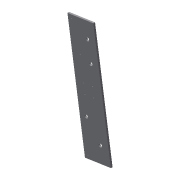
# Autodesk Inventor part: inside wall
Saved by Autodesk Inventor 2020 (Build 240168000, 168)
## iProperties
Created: 2019-10-13
Part Number: inside wall
Material: Generic
Document SubType Name: Modeling
Designer: ball
Density: 1 g/cm^3
Appearance: Default
Author: ball
Autodesk Inventor part; units mm, degrees
ref_plane "YZ Plane" through (0, 0, 0) normal (1, 0, 0) x (0, 1, 0)
ref_plane "XZ Plane" through (0, 0, 0) normal (0, 1, 0) x (-1, 0, 0)
ref_plane "XY Plane" through (0, 0, 0) normal (0, 0, 1) x (1, 0, 0)
ref_plane "Work Plane1" through (-0.0003, 0.0023, 0) normal (0, 0, 1) x (1, 0, 0)
sketch "Sketch1" plane through (-0.0003, 0.0023, 0) normal (0, 0, 1) x (1, 0, 0)
  circle A0 centre (0.0003, -0.0023) radius 6.3373 construction
  circle A1 centre (-49.0975, 326.5271) radius 6.3373 construction
  circle A2 centre (0.0003, -0.0023) radius 6.4135
  circle A3 centre (-49.0975, 326.5271) radius 6.4135
  circle A4 centre (-49.0975, 326.5271) radius 60.325 construction
  circle A5 centre (0.0003, -0.0023) radius 60.325 construction
  circle A6 centre (0.0003, -0.0023) radius 31.75 construction
  line L0 (40.3672, -54.9357) -> (-26.6702, 390.9025)
  circle A7 centre (-49.0975, 326.5271) radius 31.75 construction
  line L1 (-58.7973, -69.8464) -> (40.3672, -54.9357)
  line L2 (-125.8347, 375.9918) -> (-26.6702, 390.9025)
  circle A8 centre (-54.0299, 68.9302) radius 6.3373 construction
  circle A9 centre (-36.6118, 251.3479) radius 6.3373 construction
  circle A10 centre (-54.0299, 68.9302) radius 6.35
  circle A11 centre (-36.6118, 251.3479) radius 6.35
  line L3 (-82.6344, 131.3852) -> (-87.6899, 165.0073) construction
  line L4 (-58.7973, -69.8464) -> (-125.8347, 375.9918)
  point P0 (0.0003, -0.0023)
  dimension "d0" = 12.827
  dimension "d3" = 12.827
  dimension "d11" = 120.65
  dimension "d13" = 120.65
  dimension "d14" = 63.5
  dimension "d16" = 63.5
  dimension "d19" = 12.7
  dimension "d20" = 12.7
  constraints: 10 end point, 8 centre point, 8 coincident, 4 tangent, 3 other
  measures "d0" diameter of A2
  measures "d3" diameter of A3
  measures "d11" diameter of A4
  measures "d13" diameter of A5
  measures "d14" diameter of A6
  measures "d16" diameter of A7
  measures "d19" diameter of A10
  measures "d20" diameter of A11
extrude "Extrusion1" add sketch "Sketch1" along normal blind 6.35
sketch "Sketch2" plane through (-0.0003, 0.0023, 0) normal (0, 0, -1) x (-1, 0, 0)
  circle A0 centre (111.3879, 365.3242) radius 1.778 construction
  circle A1 centre (77.9428, 262.471) radius 1.778 construction
  circle A2 centre (31.0502, 180.1901) radius 1.778 construction
  circle A3 centre (64.857, 175.1068) radius 1.778 construction
  circle A4 centre (25.7636, 145.0307) radius 1.778 construction
  circle A5 centre (59.5704, 139.9475) radius 1.778 construction
  circle A6 centre (48.1268, -55.3992) radius 1.778 construction
  circle A7 centre (111.3879, 365.3242) radius 1.778
  circle A8 centre (77.9428, 262.471) radius 1.778
  circle A9 centre (64.857, 175.1068) radius 1.778
  circle A10 centre (59.5704, 139.9475) radius 1.778
  circle A11 centre (31.0502, 180.1901) radius 1.778
  circle A12 centre (25.7636, 145.0307) radius 1.778
  circle A13 centre (48.1268, -55.3992) radius 1.778
  point P0 (-0.0003, -0.0023)
extrude "Extrusion2" cut sketch "Sketch2" against normal through all
body "Solid1"
